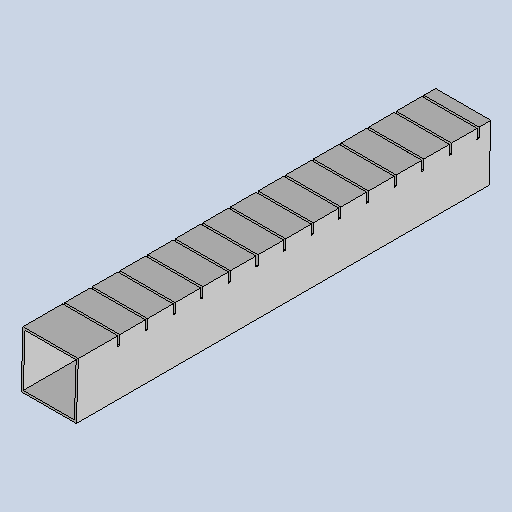
# Autodesk Inventor part: DS-B-1101 beam 24
Saved by Autodesk Inventor 2025 (Build 290162010, 162A)
## iProperties
Created: 2024-10-01
Part Number: DS-B-1101 beam 24
Material: Stainless Steel
Document SubType Name: Modeling
Designer: admin
Density: 8 g/cm^3
Appearance: Default
Author: pokla
Autodesk Inventor part; units mm, degrees
ref_plane "YZ Plane" through (0, 0, 0) normal (1, 0, 0) x (0, 1, 0)
ref_plane "XZ Plane" through (0, 0, 0) normal (0, 1, 0) x (-1, 0, 0)
ref_plane "XY Plane" through (0, 0, 0) normal (0, 0, 1) x (1, 0, 0)
sketch "Sketch1" plane through (0, 0, 0) normal (0, 1, 0) x (-1, 0, 0)
  line L0 (20, 20) -> (-20, 20)
  line L1 (-20, 20) -> (-20, -20)
  line L2 (-20, -20) -> (20, -20)
  line L3 (20, -20) -> (20, 20)
  line L4 (20, 20) -> (-20, -20) construction
  line L5 (-20, 20) -> (20, -20) construction
  line L6 (-18.5, 18.5) -> (18.5, 18.5)
  line L7 (18.5, 18.5) -> (18.5, -18.5)
  line L8 (18.5, -18.5) -> (-18.5, -18.5)
  line L9 (-18.5, -18.5) -> (-18.5, 18.5)
  point P0 (0, 0)
  dimension "d7" = 40
  dimension "d8" = 40
  dimension "d9" = 1.5
  constraints: 20 end point, 4 parallel, 2 midpoint, 2 perpendicular, 1 horizontal, 3 other
  measures "d7" distance of L2.end L1.end
  measures "d8" distance of L1.end L0.end
  measures "d9" distance between parallel lines of L0 L6
extrude "Extrusion1" add sketch "Sketch1" along normal blind 300
sketch "Sketch2" plane through (20, 0, 20) normal (1, 0, 0) x (0, 0, -1)
  line L0 (0, 0) -> (0, 300) projected
  line L1 (0, 30) -> (7, 30)
  line L2 (7, 30) -> (7, 31.5)
  line L3 (7, 31.5) -> (0, 31.5)
  line L4 (0, 31.5) -> (0, 30)
  point P0 (20, 0)
  point P1 (0, 31.5)
  dimension "d10" = 7
  dimension "d11" = 1.5
  dimension "d17" = 30
  constraints: 8 end point, 2 parallel, 1 horizontal, 1 perpendicular, 1 point on line
  measures "d10" distance of L3.end L2.end
  measures "d11" distance of L2.end L1.end
  measures "d17" distance from line of L0.start L1
extrude "Extrusion2" cut sketch "Sketch2" against normal through all
pattern_linear "Rectangular Pattern1" count 49 spacing 20 along (0, 1, 0) of "Extrusion2"
sketch "Sketch5" plane through (0, 0, 0) normal (1, 0, 0) x (0, 1, 0)
  line L0 (0, 20) -> (0, -20) projected
  line L1 (0, 20) -> (30, 20) projected
  line L2 (0, -20) -> (1.3968, 20)
  line L3 (300, -20) -> (300, 20) projected
  line L4 (300, 20) -> (298.6032, -20)
  line L5 (0, -20) -> (300, -20) projected
  point P0 (0, 0)
  dimension "d18" = 2
  dimension "d21" = 2
  constraints: 4 end point, 2 point on line
  measures "d18" angle of L2 L0
  measures "d21" angle of L3 L4
extrude "Extrusion3" cut sketch "Sketch5" along normal through all both and the other way through all
equation "\"d1\" = BEAM_4_lenth"
equation "\"d18\" = BEAM_4_angle"
equation "\"d21\" = d18"
equation "\"BEAM_4_lenth\" = 300"
equation "\"BEAM_4_angle\" = 2deg"
body "Solid1"
